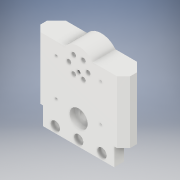
# Autodesk Inventor part: WA004
Saved by Autodesk Inventor 2017 SP1 (Build 210196100, 196)
## iProperties
Created: 2017-08-01
Part Number: WA004
Material: ABS Plastic
Document SubType Name: Modeling
Designer: Zach
Density: 1.06 g/cm^3
Appearance: CR White
Author: Zach
Autodesk Inventor part; units mm, degrees
ref_plane "YZ Plane" through (0, 0, 0) normal (1, 0, 0) x (0, 1, 0)
ref_plane "XZ Plane" through (0, 0, 0) normal (0, 1, 0) x (-1, 0, 0)
ref_plane "XY Plane" through (0, 0, 0) normal (0, 0, 1) x (1, 0, 0)
sketch "Sketch1" plane through (0, 0, 0) normal (0, 0, 1) x (1, 0, 0)
  circle A0 centre (0, 0) radius 7
  circle A1 centre (0, 65) radius 3
  line L0 (-57.25, -10) -> (57.25, -10)
  line L1 (57.25, -10) -> (57.25, 90)
  line L2 (57.25, 90) -> (-57.25, 90)
  line L3 (-57.25, 90) -> (-57.25, -10)
  line L4 (0, 65) -> (0, 0) construction
  point P0 (0, 32.5)
  point P1 (-57.25, 40)
  point P2 (0, 90)
  dimension "d0" = 14
  dimension "d1" = 6
  dimension "d2" = 65
  dimension "d3" = 114.5
  dimension "d7" = 25
  dimension "d8" = 10
  constraints: 10 end point, 3 midpoint, 2 centre point, 2 parallel, 2 vertical alignment, 1 coincident, 1 horizontal, 1 perpendicular, 1 vertical
  measures "d0" diameter of A0
  measures "d1" diameter of A1
  measures "d2" distance of L4.start point (0, 0)
  measures "d3" distance of L1.end L2.end
  measures "d7" distance from line of L2 L4.start
  measures "d8" distance from line of L0 point (0, 0)
extrude "Extrusion1" add sketch "Sketch1" along normal blind 10
sketch "Sketch2" plane through (-57.25, -10, 0) normal (0, -1, 0) x (1, 0, 0)
  line L0 (0, 10) -> (114.5, 10) projected
  line L1 (0, 10) -> (114.5, 10)
  line L2 (114.5, 10) -> (114.5, -35)
  line L3 (114.5, -35) -> (0, -35)
  line L4 (0, -35) -> (0, 10)
  point P0 (57.25, 0)
  point P1 (114.5, 0)
  dimension "d10" = 45
  constraints: 8 end point, 2 parallel, 1 horizontal, 1 perpendicular, 1 vertical alignment
  measures "d10" distance of L1.end L2.end
extrude "Extrusion2" add sketch "Sketch2" along normal blind 10
sketch "Sketch3" plane through (0, 0, 0) normal (0, 0, -1) x (-1, 0, 0)
  circle A0 centre (0, 0) radius 22.5 construction
  circle A1 centre (0, 0) radius 7 projected
  line L0 (-22.5, 0) -> (-22.5, -10)
  line L1 (57.25, -10) -> (-57.25, -10) construction
  line L2 (22.5, 0) -> (22.5, -10)
  arc A2 (22.5, 0) -> (-22.5, 0) centre (0, 0) ccw
  line L3 (-22.5, -10) -> (22.5, -10)
  dimension "d13" = 45
  constraints: 6 end point, 4 point on circle, 3 tangent, 2 centre point, 2 point on line, 1 coincident, 1 collinear, 1 parallel, 1 vertical
  measures "d13" diameter of A0
extrude "Extrusion3" add sketch "Sketch3" along normal blind 35
sketch "Sketch4" plane through (-57.25, 90, 0) normal (-1, 0, 0) x (0, 0, 1)
  line L0 (-35, -100) -> (0, -100) projected
  line L1 (-35, -100) -> (0, 0)
  line L2 (0, 0) -> (10, 0) projected
  line L3 (0, 0) -> (10, 0)
  line L4 (10, 0) -> (10, -110) projected
  line L5 (10, 0) -> (10, -110)
  line L6 (10, -110) -> (-35, -110) projected
  line L7 (10, -110) -> (-35, -110)
  line L8 (-35, -100) -> (-35, -110) projected
  line L9 (-35, -110) -> (-35, -100)
  constraints: 10 end point, 2 collinear, 2 perpendicular
extrude "Extrusion4" add sketch "Sketch4" against normal blind 10
sketch "Sketch5" plane through (57.25, 90, 10) normal (1, 0, 0) x (0, 0, -1)
  line L0 (45, -100) -> (10, 0) projected
  line L1 (10, -100) -> (10, 0) projected
  line L2 (45, -100) -> (10, -100) projected
  point P0 (0, -110)
extrude "Extrusion5" add sketch "Sketch5" against normal blind 10
sketch "Sketch9" plane through (0, 0, 0) normal (0, 0, -1) x (-1, 0, 0)
  circle A0 centre (0, 72) radius 19
  circle A1 centre (0, 65) radius 3 projected
  point P0 (0, 0)
  dimension "d28" = 38
  dimension "d95" = 7
  constraints: 1 centre point, 1 vertical alignment
  measures "d28" diameter of A0
  measures "d95" distance of A1.centre A0.centre
extrude "Extrusion8" cut sketch "Sketch9" against normal blind 1 contours A0 | A1
sketch "Sketch10" plane through (-57.25, -10, 0) normal (0, 1, 0) x (1, 0, 0)
  circle A0 centre (83.5, 20) radius 2
  line L0 (0, 0) -> (0, 35) projected
  circle A1 centre (31, 20) radius 2
  line L1 (34.75, 35) -> (79.75, 35) projected
  line L2 (34.75, 35) -> (79.75, 35) projected
  line L3 (83.5, 20) -> (31, 20)
  line L4 (79.75, 35) -> (34.75, 35) projected
  point P0 (57.25, 0)
  point P1 (114.5, 35)
  point P2 (57.25, 20)
  point P3 (57.25, 35)
  dimension "d31" = 4
  dimension "d33" = 4
  dimension "d55" = 15
  dimension "d57" = 52.5
  constraints: 2 centre point, 2 end point, 2 midpoint, 1 horizontal, 1 horizontal alignment, 1 vertical alignment
  measures "d31" diameter of A0
  measures "d33" diameter of A1
  measures "d55" distance from line of L1 L3.start
  measures "d57" distance of L3.start L3.end
extrude "Extrusion9" cut sketch "Sketch10" against normal through all
sketch "Sketch11" plane through (0, 0, -35) normal (0, 0, -1) x (-1, 0, 0)
  line L0 (57.25, -20) -> (-57.25, -20)
  line L1 (-57.25, -20) -> (-57.25, -39)
  line L2 (-57.25, -39) -> (57.25, -39)
  line L3 (57.25, -39) -> (57.25, -20)
  point P0 (0, 0)
  point P1 (57.25, -20)
  point P2 (-57.25, -20)
  point P3 (0, -20)
  dimension "d36" = 19
  constraints: 8 end point, 2 coincident, 2 parallel, 1 horizontal, 1 horizontal alignment, 1 midpoint, 1 perpendicular
  measures "d36" distance of L1.end L0.end
extrude "Extrusion10" add sketch "Sketch11" against normal blind 8.5
sketch "Sketch12" plane through (0, 0, -35) normal (0, 0, -1) x (-1, 0, 0)
  circle A0 centre (-35, -29) radius 2
  circle A1 centre (35, -29) radius 2
  line L0 (-35, -29) -> (35, -29) construction
  line L1 (-57.25, -39) -> (57.25, -39) projected
  point P0 (0, 0)
  point P1 (0, -29)
  point P2 (0, -39)
  dimension "d39" = 4
  dimension "d40" = 4
  dimension "d41" = 70
  dimension "d42" = 10
  constraints: 2 centre point, 2 end point, 2 midpoint, 1 horizontal, 1 vertical alignment
  measures "d39" diameter of A0
  measures "d40" diameter of A1
  measures "d41" distance of L0.start L0.end
  measures "d42" distance between parallel lines of L1 L0
extrude "Extrusion11" cut sketch "Sketch12" against normal through all
ref_plane "Work Plane1" through (0, 0, -6) normal (0, 0, 1) x (1, 0, 0)
sketch "Sketch14" plane through (0, 0, -6) normal (0, 0, 1) x (1, 0, 0)
  circle A0 centre (35, -29) radius 2 projected
  circle A1 centre (-35, -29) radius 2 projected
  line L0 (-57.25, -20) -> (57.25, -20) projected
  line L1 (-57.25, -20) -> (-57.25, -39) projected
  line L2 (-57.25, -39) -> (57.25, -39) projected
  line L3 (57.25, -39) -> (57.25, -20) projected
  point P0 (0, 0)
extrude "Extrusion12" add sketch "Sketch14" along normal blind 10 contours A0 | A1 | L0 L3 L2 L1
sketch "Sketch15" plane through (0, 0, 4) normal (0, 0, 1) x (1, 0, 0)
  circle A0 centre (0, -29) radius 2
  line L0 (-57.25, -39) -> (57.25, -39) projected
  point P0 (0, 0)
  point P1 (0, -39)
  dimension "d48" = 4
  dimension "d49" = 10
  constraints: 1 centre point, 1 midpoint, 1 vertical alignment
  measures "d48" diameter of A0
  measures "d49" distance from line of L0 A0.centre
extrude "Extrusion13" cut sketch "Sketch15" against normal blind 10
sketch "Sketch16" plane through (0, 0, 4) normal (0, 0, 1) x (1, 0, 0)
  circle A0 centre (0, -29) radius 2 projected
  line L0 (-57.25, -20) -> (57.25, -20) projected
  line L1 (-57.25, -20) -> (-57.25, -39) projected
  line L2 (-57.25, -39) -> (57.25, -39) projected
  line L3 (57.25, -39) -> (57.25, -20) projected
  circle A1 centre (0, -29) radius 2 projected
  circle A2 centre (0, -29) radius 7.5
  point P0 (0, 0)
  dimension "d52" = 15
  constraints: 1 centre point, 1 coincident
  measures "d52" diameter of A2
extrude "Extrusion14" add sketch "Sketch16" along normal blind 6 contours L0 L3 L2 L1
sketch "Sketch17" plane through (-57.25, -10, 0) normal (0, 1, 0) x (1, 0, 0)
  line L0 (114.5, 6) -> (0, 6) projected
  line L1 (0, 6) -> (0, 26.5) projected
  line L2 (0, 26.5) -> (114.5, 26.5) projected
  line L3 (114.5, 26.5) -> (114.5, 6) projected
  circle A0 centre (83.5, 20) radius 2 projected
  circle A1 centre (31, 20) radius 2 projected
  line L4 (0, 6) -> (0, 26.5) projected
  line L5 (0, 26.5) -> (-36.5, -10) construction
  line L6 (0, 26.5) -> (51.6188, 26.5) construction
  line L7 (114.5, -10) -> (0, -10) projected
  line L8 (0, -10) -> (-36.5, -10) construction
  line L9 (0, 26.5) -> (0, -10)
  line L10 (114.5, 26.5) -> (114.5, 6) projected
  line L11 (114.5, 26.5) -> (151, -10) construction
  line L12 (114.5, -10) -> (151, -10) construction
  line L13 (114.5, -10) -> (114.5, 26.5)
  line L14 (129.5, 11.5) -> (129.5, -10)
  line L15 (114.5, 26.5) -> (129.5, 11.5)
  line L16 (129.5, -10) -> (114.5, -10)
  line L17 (-15, 11.5) -> (-15, -10)
  line L18 (0, 35) -> (0, 26.5) projected
  line L19 (0, 26.5) -> (-15, 11.5)
  line L20 (0, -10) -> (-15, -10)
  point P0 (57.25, 0)
  dimension "d58" = 135
  dimension "d60" = 135
  dimension "d65" = 15
  dimension "d66" = 15
  constraints: 26 end point, 4 point on line, 3 collinear, 3 horizontal, 3 perpendicular, 1 equal length
  measures "d58" angle of L5 L6
  measures "d60" angle of L11 L2
  measures "d65" distance between parallel lines of L13 L14
  measures "d66" distance between parallel lines of L9 L17
extrude "Extrusion15" add sketch "Sketch17" along normal blind 100 contours L3 L15 L14 L16 L13 | L9 L20 L17 L19 L1
sketch "Sketch18" plane through (57.25, 14.2857, -26.5) normal (-1, 0, 0) x (0, 0, 1)
  line L0 (26.5, 75.7143) -> (-8.5, -24.2857) construction
  line L1 (26.5, -24.2857) -> (-8.5, -24.2857) construction
  line L2 (26.5, 75.7143) -> (26.5, -24.2857) construction
  line L3 (-8.5, -24.2857) -> (-8.5, 75.7143)
  line L4 (-8.5, 75.7143) -> (26.5, 75.7143)
  line L5 (-8.5, -24.2857) -> (26.5, 75.7143)
  constraints: 6 end point, 1 collinear, 1 perpendicular, 1 vertical
extrude "Extrusion16" cut sketch "Sketch18" along normal through all both and the other way through all
sketch "Sketch21" plane through (-47.25, 90, 0) normal (0, 1, 0) x (1, 0, 0)
  line L0 (-25, -10) -> (-10, -10) projected
  line L1 (-25, -10) -> (-19.6967, -4.6967) construction
  line L2 (-25, -10) -> (-17.5, -10) construction
  line L3 (-25, 11.5) -> (-25, -10) projected
  line L4 (-25, 0.6066) -> (-14.3934, -10)
  line L5 (-25, 0.6066) -> (-25, -10)
  line L6 (-14.3934, -10) -> (-25, -10)
  line L7 (-25, -10) -> (119.5, -10) projected
  line L8 (119.5, -10) -> (114.1967, -4.6967) construction
  line L9 (119.5, -10) -> (127, -10) construction
  line L10 (108.8934, -10) -> (119.5, 0.6066)
  line L11 (119.5, -10) -> (119.5, 11.5) projected
  line L12 (108.8934, -10) -> (123.8934, -10) construction
  line L13 (108.8934, -10) -> (119.5, -10)
  line L14 (119.5, -10) -> (119.5, 0.6066)
  point P0 (47.25, 0)
  dimension "d75" = 7.5
  dimension "d76" = 45
  dimension "d77" = 7.5
  dimension "d78" = 135
  dimension "d79" = 45
  constraints: 22 end point, 4 point on line, 3 equal length, 3 horizontal, 2 collinear, 2 midpoint, 1 vertical
  measures "d75" distance of L1.end L0.start
  measures "d76" angle of L2 L1
  measures "d77" distance of L7.end L8.end
  measures "d78" angle of L9 L8
  measures "d79" angle of L12 L10
extrude "Extrusion19" cut sketch "Sketch21" against normal through all
sketch "Sketch22" plane through (0, 0, 10) normal (0, 0, 1) x (1, 0, 0)
  circle A0 centre (0, 0) radius 14.5
  circle A1 centre (0, 0) radius 7 projected
  dimension "d82" = 29
  constraints: 1 centre point, 1 coincident
  measures "d82" diameter of A0
extrude "Extrusion20" cut sketch "Sketch22" against normal blind 9
sketch "Sketch23" plane through (-47.25, -10, -35) normal (0, 0, -1) x (-1, 0, 0)
  circle A0 centre (-47.25, 10) radius 7 projected
  circle A1 centre (-47.25, 10) radius 14.5
  dimension "d85" = 29
  constraints: 1 centre point, 1 coincident
  measures "d85" diameter of A1
extrude "Extrusion21" cut sketch "Sketch23" against normal blind 16.5
sketch "Sketch24" plane through (0, 72, 1) normal (0, 0, -1) x (-1, 0, 0)
  circle A0 centre (0, -7) radius 3 projected
  circle A1 centre (0, -7) radius 6.5
  point P0 (0, -72)
  dimension "d88" = 13
  constraints: 1 centre point, 1 coincident
  measures "d88" diameter of A1
extrude "Extrusion22" cut sketch "Sketch24" against normal blind 7
sketch "Sketch27" plane through (0, 0, 1) normal (0, 0, -1) x (-1, 0, 0)
  arc A0 (-6.0828, 90) -> (6.0828, 90) centre (0, 72) ccw construction
  circle A1 centre (15.5, 72) radius 2
  circle A2 centre (7.75, 85.4234) radius 2
  circle A3 centre (-7.75, 85.4234) radius 2
  circle A4 centre (-15.5, 72) radius 2
  circle A5 centre (-7.75, 58.5766) radius 2
  circle A6 centre (7.75, 58.5766) radius 2
  point P0 (0, 0)
  dimension "d96" = 4
  dimension "d97" = 15.5
  dimension "d100" = 360
  constraints: 6 centre point, 1 horizontal alignment, 13 other
  measures "d96" diameter of A1
  measures "d97" distance of A0.centre A1.centre
extrude "Extrusion24" cut sketch "Sketch27" against normal blind 10
sketch "Sketch28" plane through (0, 0, 10) normal (0, 0, 1) x (1, 0, 0)
  circle A0 centre (-7.75, 85.4234) radius 2 projected
  circle A1 centre (7.75, 85.4234) radius 2 projected
  circle A2 centre (15.5, 72) radius 2 projected
  circle A3 centre (7.75, 58.5766) radius 2 projected
  circle A4 centre (-7.75, 58.5766) radius 2 projected
  circle A5 centre (-15.5, 72) radius 2 projected
  circle A6 centre (15.5, 72) radius 3.5
  arc A7 (-6.0828, 90) -> (6.0828, 90) centre (0, 72) ccw construction
  circle A8 centre (7.75, 85.4234) radius 3.5
  circle A9 centre (-7.75, 85.4234) radius 3.5
  circle A10 centre (-15.5, 72) radius 3.5
  circle A11 centre (-7.75, 58.5766) radius 3.5
  circle A12 centre (7.75, 58.5766) radius 3.5
  point P0 (0, 0)
  dimension "d104" = 7
  dimension "d107" = 360
  constraints: 6 centre point, 6 coincident, 19 other
  measures "d104" diameter of A6
extrude "Extrusion25" cut sketch "Sketch28" against normal blind 3 contours A0 | A1 | A2 | A3 | A4 | A5 | A6 | A8 | A9 | A10 | A11 | A12
sketch "Sketch29" plane through (0, 0, 0) normal (0, 0, -1) x (-1, 0, 0)
  arc A0 (-6.0828, 90) -> (6.0828, 90) centre (0, 72) ccw projected
  arc A1 (-12.6408, 98.1) -> (12.6408, 98.1) centre (0, 72) ccw construction
  line L0 (-6.0828, 90) -> (-22.7376, 90)
  line L1 (61.6434, 90) -> (-61.6434, 90) construction
  line L2 (6.0828, 90) -> (22.7376, 90)
  arc A2 (-22.7376, 90) -> (22.7376, 90) centre (0, 72) ccw
  point P0 (0, 0)
  dimension "d111" = 10
  constraints: 6 point on circle, 4 end point, 2 centre point, 2 concentric, 2 point on line
  measures "d111" radial gap between concentric circles of A0 A1
extrude "Extrusion26" add sketch "Sketch29" along normal blind 35
sketch "Sketch31" plane through (-57.25, -10, 0) normal (0, -1, 0) x (1, 0, 0)
  line L0 (104.5, 0) -> (104.5, -35) projected
  line L1 (114.5, -26.5) -> (114.5, -35) projected
  line L2 (114.5, -26.5) -> (129.5, -11.5) projected
  line L3 (129.5, -11.5) -> (129.5, -0.6066) projected
  line L4 (118.8934, 10) -> (128.8934, 0) projected
  line L5 (10, -35) -> (10, 0) projected
  line L6 (0, -26.5) -> (0, -35) projected
  line L7 (-15, -11.5) -> (0, -26.5) projected
  line L8 (-15, -0.6066) -> (-15, -11.5) projected
  line L9 (-14.3934, 0) -> (-4.3934, 10) projected
  line L10 (-4.3934, 10) -> (118.8934, 10) construction
  line L11 (114.5, -35) -> (104.5, -35)
  line L12 (104.5, 0) -> (104.5, 10)
  line L13 (10, -35) -> (0, -35)
  line L14 (10, 0) -> (10, 10)
  line L15 (118.8934, 10) -> (104.5, 10)
  line L16 (-4.3934, 10) -> (10, 10)
  line L17 (10, 0) -> (-14.3934, 0) construction
  line L18 (-14.3934, 0) -> (-15, -0.6066)
  line L19 (129.5, -0.6066) -> (128.8934, 0)
  point P0 (57.25, 0)
  constraints: 16 end point, 2 collinear, 2 horizontal, 2 perpendicular, 2 point on line
extrude "Extrusion27" add sketch "Sketch31" against normal blind 100
sketch "Sketch33" plane through (0, 0, -6) normal (0, 0, -1) x (-1, 0, 0)
  circle A0 centre (0, -29) radius 2 projected
  line L0 (57.25, -39) -> (57.25, -20) projected
  line L1 (-57.25, -20) -> (57.25, -20) projected
  line L2 (-57.25, -20) -> (-57.25, -39) projected
  line L3 (-57.25, -39) -> (57.25, -39) projected
  point P0 (0, 0)
extrude "Extrusion28" cut sketch "Sketch33" along normal through all contours A0 | L3 L2 L1 L0
sketch "Sketch34" plane through (-57.25, -10, -26.5) normal (-0.7071068, 0, -0.7071068) x (-0.7071068, 0, 0.7071068)
  line L0 (10.6066, 80) -> (10.6066, 20) construction
  line L1 (21.2132, 0) -> (21.2132, 100) construction
  line L2 (0, 100) -> (21.2132, 100) construction
  circle A0 centre (10.6066, 80) radius 1.5
  circle A1 centre (10.6066, 20) radius 1.5
  point P0 (-21.7435, 10)
  point P1 (10.6066, 50)
  point P2 (10.6066, 100)
  point P3 (21.2132, 50)
  dimension "d118" = 60
  dimension "d119" = 3
  dimension "d120" = 3
  constraints: 3 midpoint, 2 centre point, 2 coincident, 2 end point, 1 horizontal alignment, 1 vertical, 1 vertical alignment
  measures "d118" distance of L0.start L0.end
  measures "d119" diameter of A0
  measures "d120" diameter of A1
extrude "Extrusion29" cut sketch "Sketch34" against normal through all
sketch "Sketch35" plane through (72.25, -10, -11.5) normal (0.7071068, 0, -0.7071068) x (-0.7071068, 0, -0.7071068)
  line L0 (10.6066, 80) -> (10.6066, 20) construction
  line L1 (0, 0) -> (0, 100) construction
  line L2 (0, 100) -> (21.2132, 100) construction
  circle A0 centre (10.6066, 80) radius 1.5
  circle A1 centre (10.6066, 20) radius 1.5
  point P0 (42.9567, 10)
  point P1 (10.6066, 100)
  point P2 (10.6066, 50)
  point P3 (0, 50)
  dimension "d123" = 60
  dimension "d124" = 3
  dimension "d125" = 3
  constraints: 3 midpoint, 2 centre point, 2 coincident, 2 end point, 1 horizontal alignment, 1 vertical, 1 vertical alignment
  measures "d123" distance of L0.start L0.end
  measures "d124" diameter of A0
  measures "d125" diameter of A1
extrude "Extrusion30" cut sketch "Sketch35" against normal through all
sketch "Sketch36" plane through (0, 0, 0) normal (0, 0, -1) x (-1, 0, 0)
  line L0 (-47.25, 90) -> (-22.7376, 90)
  line L1 (-22.7376, 90) -> (-22.7376, 80)
  line L2 (-22.7376, 80) -> (-47.25, 80)
  line L3 (-47.25, 80) -> (-47.25, 90)
  line L4 (22.7376, 90) -> (47.25, 90) projected
  line L5 (47.25, 90) -> (22.7376, 90)
  line L6 (22.7376, 90) -> (22.7376, 80)
  line L7 (22.7376, 80) -> (47.25, 80)
  line L8 (47.25, 80) -> (47.25, 90)
  line L9 (22.7376, 90) -> (6.0828, 90) projected
  line L10 (-5, 43.4343) -> (5, 43.4343)
  line L11 (5, 43.4343) -> (5, 21.9374)
  line L12 (5, 21.9374) -> (-5, 21.9374)
  line L13 (-5, 21.9374) -> (-5, 43.4343)
  line L14 (-6.0828, 90) -> (6.0828, 90) projected
  arc A0 (-22.7376, 90) -> (22.7376, 90) centre (0, 72) ccw projected
  arc A1 (22.5, 0) -> (-22.5, 0) centre (0, 0) ccw projected
  point P0 (0, 43.4343)
  point P1 (0, 90)
  dimension "d128" = 10
  dimension "d129" = 10
  dimension "d130" = 10
  constraints: 24 end point, 6 parallel, 3 horizontal, 3 perpendicular, 3 vertical alignment, 2 midpoint, 2 point on circle
  measures "d128" distance of L0.end L1.end
  measures "d129" distance of L5.end L6.end
  measures "d130" distance of L11.end L12.end
extrude "Extrusion31" add sketch "Sketch36" along normal blind 35
sketch "Sketch37" plane through (0, 0, 0) normal (0, 0, -1) x (-1, 0, 0)
  line L0 (47.25, 11.0607) -> (47.25, 68.9393) projected
  line L1 (-47.25, -10) -> (-47.25, 80) projected
  line L2 (47.25, 21.9374) -> (-47.25, 21.9374)
  line L3 (-47.25, 21.9374) -> (-47.25, 31.9374)
  line L4 (-47.25, 31.9374) -> (47.25, 31.9374)
  line L5 (47.25, 31.9374) -> (47.25, 21.9374)
  line L6 (47.25, -10) -> (47.25, 80) projected
  point P0 (0, 0)
  point P1 (5, 21.9374)
  dimension "d133" = 10
  constraints: 8 end point, 4 point on line, 2 parallel, 1 horizontal, 1 perpendicular
  measures "d133" distance between parallel lines of L4 L2
extrude "Extrusion32" add sketch "Sketch37" along normal blind 35
sketch "Sketch38" plane through (0, 0, 10) normal (0, 0, 1) x (1, 0, 0)
  line L0 (-37.5, -29) -> (37.5, -29) construction
  circle A0 centre (0, -29) radius 2 projected
  circle A1 centre (37.5, -29) radius 1.5
  circle A2 centre (-37.5, -29) radius 1.5
  point P0 (0, 0)
  point P1 (0, -29)
  dimension "d136" = 75
  dimension "d137" = 3
  dimension "d138" = 3
  constraints: 3 coincident, 2 centre point, 2 end point, 1 horizontal, 1 midpoint
  measures "d136" distance of L0.start L0.end
  measures "d137" diameter of A1
  measures "d138" diameter of A2
extrude "Extrusion33" cut sketch "Sketch38" against normal through all
sketch "Sketch39" plane through (0, 0, 10) normal (0, 0, 1) x (1, 0, 0)
  circle A0 centre (37.5, -29) radius 1.5 projected
  circle A1 centre (-37.5, -29) radius 1.5 projected
  circle A2 centre (-37.5, -29) radius 7.5
  circle A3 centre (37.5, -29) radius 7.5
  point P0 (0, 0)
  dimension "d141" = 15
  dimension "d142" = 15
  constraints: 2 centre point, 2 coincident
  measures "d141" diameter of A2
  measures "d142" diameter of A3
extrude "Extrusion34" cut sketch "Sketch39" against normal blind 6 contours A0 | A1 | A2 | A3
sketch "Sketch40" plane through (0, 0, 0) normal (0, 0, -1) x (-1, 0, 0)
  arc A0 (10.5, -10) -> (-10.5, -10) centre (0, 0) ccw projected
  arc A1 (22.5, 0) -> (5, 21.9374) centre (0, 0) ccw projected
  arc A2 (-5, 21.9374) -> (-22.5, 0) centre (0, 0) ccw projected
  line L0 (-22.5, -10) -> (-22.5, 0) projected
  line L1 (-10.5, -10) -> (-22.5, -10) projected
  line L2 (22.5, -10) -> (10.5, -10) projected
  line L3 (22.5, 0) -> (22.5, -10) projected
  arc A3 (-10.5, -10) -> (10.5, -10) centre (0, 0) ccw projected
  line L4 (5, 21.9374) -> (-5, 21.9374) projected
  arc A4 (-5, 21.9374) -> (-22.5, 0) centre (0, 0) ccw projected
  line L5 (-22.5, -10) -> (-22.5, 0) projected
  line L6 (-10.5, -10) -> (-22.5, -10) projected
  arc A5 (10.5, -10) -> (-10.5, -10) centre (0, 0) ccw projected
  line L7 (22.5, -10) -> (10.5, -10) projected
  line L8 (22.5, 0) -> (22.5, -10) projected
  arc A6 (22.5, 0) -> (5, 21.9374) centre (0, 0) ccw projected
extrude "Extrusion35" add sketch "Sketch40" along normal blind 35 contours A0 L1 L0 A2 L4 A1 L3 L2
sketch "Sketch41" plane through (57.25, -20, -35) normal (0, 0, -1) x (-1, 0, 0)
  circle A0 centre (57.25, 20) radius 14.5 projected
  line L0 (10, 10) -> (34.75, 10) projected
  line L1 (10, 10) -> (10, 41.9374) projected
  line L2 (10, 41.9374) -> (52.25, 41.9374) projected
  arc A1 (52.25, 41.9374) -> (34.75, 20) centre (57.25, 20) ccw projected
  line L3 (34.75, 20) -> (34.75, 10) projected
  line L4 (10, 51.9374) -> (10, 100) projected
  line L5 (10, 100) -> (29.3753, 100) projected
  arc A2 (29.3753, 100) -> (52.25, 63.4343) centre (57.25, 92) ccw projected
  line L6 (52.25, 63.4343) -> (52.25, 51.9374) projected
  line L7 (52.25, 51.9374) -> (10, 51.9374) projected
  line L8 (62.25, 51.9374) -> (62.25, 63.4343) projected
  arc A3 (62.25, 63.4343) -> (85.1247, 100) centre (57.25, 92) ccw projected
  line L9 (85.1247, 100) -> (104.5, 100) projected
  line L10 (104.5, 51.9374) -> (104.5, 100) projected
  line L11 (104.5, 51.9374) -> (62.25, 51.9374) projected
  line L12 (79.75, 10) -> (79.75, 20) projected
  arc A4 (79.75, 20) -> (62.25, 41.9374) centre (57.25, 20) ccw projected
  line L13 (62.25, 41.9374) -> (104.5, 41.9374) projected
  line L14 (104.5, 10) -> (104.5, 41.9374) projected
  line L15 (79.75, 10) -> (104.5, 10) projected
  line L16 (0, 110) -> (51.1672, 110) projected
  line L17 (0, 0) -> (0, 110) projected
  line L18 (0, 0) -> (114.5, 0) projected
  line L19 (114.5, 0) -> (114.5, 110) projected
  line L20 (114.5, 110) -> (63.3328, 110) projected
  arc A5 (51.1672, 110) -> (63.3328, 110) centre (57.25, 92) ccw projected
extrude "Extrusion36" cut sketch "Sketch41" against normal blind 8.5
sketch "Sketch42" plane through (57.25, -20, -26.5) normal (0, 0, -1) x (-1, 0, 0)
  arc A0 (51.1672, 110) -> (63.3328, 110) centre (57.25, 92) ccw projected
  arc A1 (62.25, 63.4343) -> (85.1247, 100) centre (57.25, 92) ccw projected
  circle A2 centre (57.25, 92) radius 29
  circle A3 centre (57.25, 92) radius 19
  point P0 (57.25, 20)
  constraints: 2 centre point, 2 coincident, 2 concentric
extrude "Extrusion37" add sketch "Sketch42" against normal blind 36.5
sketch "Sketch43" plane through (0, 0, 1) normal (0, 0, -1) x (-1, 0, 0)
  line L0 (-6.0828, 90) -> (6.0828, 90) projected
  arc A0 (6.0828, 90) -> (-6.0828, 90) centre (0, 72) ccw
  circle A1 centre (0, 72) radius 19 construction
  arc A2 (6.0828, 90) -> (-6.0828, 90) centre (0, 72) ccw projected
  point P0 (0, 0)
  constraints: 2 point on circle, 1 centre point, 1 concentric
extrude "Extrusion38" add sketch "Sketch43" against normal blind 9
body "Solid1"
